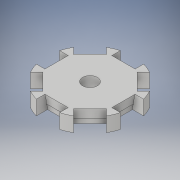
# Autodesk Inventor part: Restraining_cylinder
Saved by Autodesk Inventor 2019 (Build 230136000, 136)
## iProperties
Created: 2019-12-17
Part Number: Restraining_cylinder
Material: Generic
Document SubType Name: Modeling
Designer: Jorian Brusind
Density: 1 g/cm^3
Appearance: Default
Author: Jorian Brusind
Autodesk Inventor part; units mm, degrees
ref_plane "YZ Plane" through (0, 0, 0) normal (1, 0, 0) x (0, 1, 0)
ref_plane "XZ Plane" through (0, 0, 0) normal (0, 1, 0) x (-1, 0, 0)
ref_plane "XY Plane" through (0, 0, 0) normal (0, 0, 1) x (1, 0, 0)
sketch "Sketch1" plane through (0, 0, 0) normal (0, 1, 0) x (-1, 0, 0)
  circle A0 centre (0, 0) radius 15
  dimension "d0" = 30
  constraints: 1 centre point, 1 coincident
  measures "d0" diameter of A0
extrude "Extrusion1" add sketch "Sketch1" along normal blind 5
sketch "Sketch2" plane through (0, 0, 0) normal (0, 0, 1) x (1, 0, 0)
  line L0 (14.9712, 4.1722) -> (14.6226, 0.1874)
  line L1 (14.9712, 4.1722) -> (12.9712, 7.6363) construction
  circle A0 centre (14.6226, 0.1874) radius 1.75
  circle A1 centre (14.6226, 0.1874) radius 4
  line L2 (10.9974, 1.8779) -> (7.443, 8.0342) construction
  line L3 (18.5658, -0.4842) -> (16.5658, 2.9799) construction
  line L4 (18.5658, -0.4842) -> (17.5658, 1.2478) construction
  line L5 (10.9974, 1.8779) -> (5.9974, 10.5381) construction
  spline S0 degree 2 poles (10.9974, 1.8779) (11.3822, 8.759) (18.145, 14.8014) knots 0 0 0 1 1 1
  spline S1 degree 2 poles (18.5658, -0.4842) (18.7234, 6.6355) (20.6064, 13.9931) knots 0 0 0 1 1 1
  line L6 (20.6064, 13.9931) -> (18.145, 14.8014)
  point P0 (0, 0)
  point P1 (15, 0)
  point P2 (15, 5)
  point P3 (14.9712, 4.1722)
  point P4 (12.7212, 8.0706)
  point P5 (19.1384, 6.5778)
  dimension "d25" = 4
  dimension "d26" = 145
  dimension "d27" = 3.5
  constraints: 14 end point, 3 point on circle, 2 centre point, 2 coincident, 1 equal length, 6 other
  measures "d25" distance of L0.start L0.end
  measures "d26" angle of L1 L0
  measures "d27" diameter of A0
sketch "Sketch3" plane through (0, 5, 0) normal (0, 1, 0) x (1, 0, 0)
  circle A0 centre (0, 0) radius 2.55
  dimension "d9" = 5.1
  constraints: 1 centre point, 1 coincident
  measures "d9" diameter of A0
hole "Hole1" at (0, 5, 0) direction (0, -1, 0) diameter 3.8 end through all counterbore diameter 5.1 counterbore depth 3.8
extrude "Extrusion4" cut sketch "Sketch2" along normal mid plane 8 contours A0 | A1 S1 | A1 S0 L6 S1 picked at (17.8462, 0.1045)
pattern_circular "Circular Pattern3" count 8 over 360 about axis through (0, 3.1, 0) along (0, 1, 0) of "Extrusion4"
body "Solid1"
